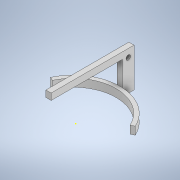
# Autodesk Inventor part: dynamicGripper
Saved by Autodesk Inventor 2020 (Build 240168000, 168)
## iProperties
Created: 2023-01-18
Part Number: dynamicGripper
Material: Generic
Document SubType Name: Modeling
Designer: legoo
Density: 1 g/cm^3
Appearance: Default
Author: legoo
## iProperties of the stored document _3DPrint.ipt
Created: 2023-01-18
Part Number: _3DPrint
Material: Generic
Document SubType Name: Modeling
Designer: legoo
Density: 1 g/cm^3
Appearance: Default
Author: legoo
Autodesk Inventor part; units mm, degrees
ref_plane "YZ Plane" through (0, 0, 0) normal (1, 0, 0) x (0, 1, 0)
ref_plane "XZ Plane" through (0, 0, 0) normal (0, 1, 0) x (-1, 0, 0)
ref_plane "XY Plane" through (0, 0, 0) normal (0, 0, 1) x (1, 0, 0)
sketch "Sketch1" plane through (0, 0, 0) normal (0, 1, 0) x (-1, 0, 0)
  arc A0 (-29.9263, -13.9549) -> (29.9263, -13.9549) centre (0, 0) ccw
  arc A1 (-32.6452, -15.2227) -> (32.6452, -15.2227) centre (0, 0) ccw
  line L0 (54.2691, 0) -> (-55.7933, 0) construction
  line L1 (29.9263, -13.9549) -> (32.6452, -15.2227)
  line L2 (-29.9263, -13.9549) -> (-32.6452, -15.2227)
  dimension "d0" = 66.04
  dimension "d1" = 3
  dimension "d2" = 25
  dimension "d3" = 25
  constraints: 6 end point, 4 point on circle, 2 centre point, 1 coincident, 1 horizontal
  measures "d0" diameter of A0
  measures "d1" radial gap between concentric circles of A0 A1
  measures "d2" angle of L0 L1
  measures "d3" angle of L0 L2
extrude "Extrusion1" add sketch "Sketch1" along normal blind 6
sketch "Sketch2" plane through (0, 0, 0) normal (0, -1, 0) x (1, 0, 0)
  arc A0 (-32.6452, -15.2227) -> (32.6452, -15.2227) centre (0, 0) ccw projected
  line L0 (2, -35.9644) -> (2, -44.9644)
  line L1 (2, -44.9644) -> (-2, -44.9644)
  line L2 (-2, -44.9644) -> (-2, -35.9644)
  dimension "d6" = 9
  dimension "d7" = 2
  dimension "d8" = 2
  constraints: 6 end point, 2 perpendicular, 2 point on circle, 1 vertical
  measures "d6" distance of L0.start L0.end
  measures "d7" distance from line of L0 point (0, 0)
  measures "d8" distance from line of point (0, 0) L2
extrude "Extrusion2" add sketch "Sketch2" against normal blind 30
sketch "Sketch3" plane through (2, 0, -35.9644) normal (1, 0, 0) x (0, 0, -1)
  circle A0 centre (4.5, 24) radius 1.75
  line L0 (9, 0) -> (9, 30) projected
  line L1 (0, 30) -> (9, 30) projected
  line L2 (9, 0) -> (0, 0) projected
  point P0 (-35.9644, 0)
  dimension "d11" = 3.5
  dimension "d12" = 4.5
  dimension "d16" = 24
  constraints: 1 centre point
  measures "d11" diameter of A0
  measures "d12" distance from line of L0 A0.centre
  measures "d16" distance from line of L2 A0.centre
extrude "Extrusion3" cut sketch "Sketch3" against normal blind 26
sketch "Sketch5" plane through (0, 30, 0) normal (0, 1, 0) x (1, 0, 0)
  line L0 (-2, 44.9644) -> (-2, 35.9644) projected
  line L1 (-2, 35.9644) -> (-2, -19.0356)
  line L2 (-2, -19.0356) -> (2, -19.0356)
  line L3 (2, -19.0356) -> (2, 35.9644)
  arc A0 (2, 35.9644) -> (-2, 35.9644) centre (0, 0) ccw projected
  dimension "d22" = 55
  constraints: 6 end point, 1 collinear, 1 parallel, 1 perpendicular
  measures "d22" distance of L0.end L1.end
extrude "Extrusion5" add sketch "Sketch5" against normal blind 5
sketch "Sketch6" plane through (2, 0, -35.9644) normal (1, 0, 0) x (0, 0, -1)
  point P0 (-35.9644, 0)
body "Solid1"
